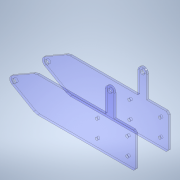
# Autodesk Inventor part: Papa John Mounting Plate with hinge half 1
Saved by Autodesk Inventor 2020 (Build 240168000, 168)
## iProperties
Created: 2020-01-31
Part Number: Papa John Mounting Plate with hinge half 1
Material: Polycarbonate, Clear
Document SubType Name: Modeling
Designer: aidan
Density: 1.2 g/cm^3
Appearance: Polycarbonate - Clear
Author: aidan
Autodesk Inventor part; units mm, degrees
ref_plane "YZ Plane" through (0, 0, 0) normal (1, 0, 0) x (0, 1, 0)
ref_plane "XZ Plane" through (0, 0, 0) normal (0, 1, 0) x (-1, 0, 0)
ref_plane "XY Plane" through (0, 0, 0) normal (0, 0, 1) x (1, 0, 0)
sketch "Sketch1" plane through (0, 0, 0) normal (0, 0, 1) x (1, 0, 0)
  line L0 (0, 0) -> (44.45, 0) construction
  line L1 (44.45, 0) -> (44.45, -25.4) construction
  line L2 (44.45, -25.4) -> (0, -25.4) construction
  line L3 (0, -25.4) -> (0, 0) construction
  line L4 (-88.9, 12.7) -> (57.15, 12.7)
  line L5 (57.15, 12.7) -> (57.15, -38.1)
  line L6 (57.15, -38.1) -> (-88.9, -38.1)
  line L7 (-88.9, 12.7) -> (-132.8941, -12.7)
  line L8 (-132.8941, -12.7) -> (-88.9, -38.1)
  line L9 (-88.9, 12.7) -> (-88.9, -38.1) construction
  dimension "d0" = 44.45
  dimension "d1" = 25.4
  dimension "d2" = 12.7
  dimension "d3" = 12.7
  dimension "d5" = 12.7
  dimension "d37" = 146.05
  dimension "d38" = 50.8
  constraints: 20 end point, 3 parallel, 2 horizontal, 2 perpendicular, 1 coincident, 1 equal length, 1 vertical
  measures "d0" distance of L0.start L0.end
  measures "d1" distance of L0.end L1.end
  measures "d2" distance between parallel lines of L4 L0
  measures "d3" distance between parallel lines of L6 L2
  measures "d5" distance between parallel lines of L5 L1
  measures "d37" distance of L4.start L4.end
  measures "d38" distance of L4.start L7.end
extrude "Extrusion1" add sketch "Sketch1" along normal blind 2.9972
sketch "Sketch2" plane through (0, 0, 2.9972) normal (0, 0, 1) x (1, 0, 0)
  line L0 (0, -25.4) -> (44.45, -25.4) construction
  line L1 (44.45, -25.4) -> (44.45, 0) construction
  line L2 (44.45, 0) -> (0, 0) construction
  line L3 (0, 0) -> (0, -25.4) construction
  line L4 (-88.9, -38.1) -> (57.15, -38.1) projected
  line L5 (57.15, -38.1) -> (57.15, 12.7) projected
  circle A0 centre (0, 0) radius 2.0193
  circle A1 centre (44.45, 0) radius 2.0193
  circle A2 centre (44.45, -25.4) radius 2.0193
  circle A3 centre (0, -25.4) radius 2.0193
  point P0 (0, 0)
  dimension "d8" = 12.7
  dimension "d9" = 25.4
  dimension "d10" = 12.7
  dimension "d11" = 44.45
  dimension "d12" = 4.0386
  constraints: 8 end point, 4 centre point, 4 coincident, 3 equal radius, 2 parallel, 1 horizontal, 1 perpendicular
  measures "d8" distance between parallel lines of L4 L0
  measures "d9" distance of L0.end L1.end
  measures "d10" distance between parallel lines of L5 L1
  measures "d11" distance of L1.end L2.end
  measures "d12" diameter of A0
extrude "Extrusion2" cut sketch "Sketch2" against normal through all
fillet "Fillet1" radius 6.35 1 edges at (-132.8941, -12.7, 1.4986)
chamfer "Chamfer1" distance 3.175 angle 45 4 edges at (57.15, 12.7, 1.4986) (57.15, -38.1, 1.4986) (-88.9, 12.7, 1.4986) (-88.9, -38.1, 1.4986)
sketch "Sketch3" plane through (0, 0, 2.9972) normal (0, 0, 1) x (1, 0, 0)
  arc A0 (-123.3691, -7.2007) -> (-123.3691, -18.1993) centre (-120.1941, -12.7) ccw projected
  circle A1 centre (-120.1941, -12.7) radius 3.175
  point P0 (0, 0)
  dimension "d19" = 6.35
  constraints: 1 centre point, 1 coincident
  measures "d19" diameter of A1
hole "Hole1" at (-120.1941, -12.7, 2.9972) direction (0, 0, -1) diameter 6.35 end through all
sketch "Sketch4" plane through (0, 0, 2.9972) normal (0, 0, 1) x (1, 0, 0)
  circle A0 centre (19.05, 44.45) radius 3.175
  line L0 (53.975, 12.7) -> (-85.725, 12.7) projected
  line L1 (12.7, 12.7) -> (25.4, 12.7)
  line L2 (25.4, 12.7) -> (25.4, 50.8)
  line L3 (25.4, 50.8) -> (12.7, 50.8)
  line L4 (12.7, 50.8) -> (12.7, 12.7)
  line L5 (57.15, -34.925) -> (57.15, 9.525) projected
  point P0 (0, 0)
  dimension "d27" = 6.35
  dimension "d28" = 6.35
  dimension "d29" = 12.7
  dimension "d30" = 6.35
  dimension "d31" = 31.75
  dimension "d32" = 38.1
  constraints: 8 end point, 2 parallel, 1 centre point, 1 horizontal, 1 perpendicular, 1 point on line
  measures "d27" diameter of A0
  measures "d28" distance from line of L3 A0.centre
  measures "d29" distance between parallel lines of L2 L4
  measures "d30" distance from line of L2 A0.centre
  measures "d31" distance between parallel lines of L2 L5
  measures "d32" distance of L3.end L1.start
extrude "Extrusion3" add sketch "Sketch4" against normal blind 2.9972
fillet "Fillet2" radius 6.35 2 edges at (12.7, 50.8, 1.4986) (25.4, 50.8, 1.4986)
ref_plane "Work Plane1" through (0, 0, 25.2222) normal (0, 0, 1) x (1, 0, 0)
mirror "Mirror1" about plane through (0, 0, 25.2222) normal (0, 0, 1) of "Extrusion1", "Extrusion2", "Fillet1", "Chamfer1", "Hole1", "Extrusion3", "Fillet2"
body "Solid1"
